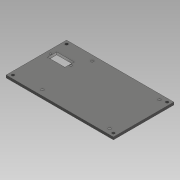
# Autodesk Inventor part: 基本板上
Saved by Autodesk Inventor 2017 (Build 210142000, 142)
## iProperties
Part Number: 基本板上
Material: 一般
Document SubType Name: Modeling
Designer: HISAAKI
Density: 1 g/cm^3
Appearance: 既定
Mass: 37.3682 g
Surface Area: 242.536 cm^2
Volume: 37.3682 cm^3
Author: HISAAKI
Autodesk Inventor part; units mm, degrees
ref_plane "YZ Plane" through (0, 0, 0) normal (1, 0, 0) x (0, 1, 0)
ref_plane "XZ Plane" through (0, 0, 0) normal (0, 1, 0) x (-1, 0, 0)
ref_plane "XY Plane" through (0, 0, 0) normal (0, 0, 1) x (1, 0, 0)
sketch "スケッチ1" plane through (0, 0, 0) normal (0, 0, 1) x (1, 0, 0)
  line L0 (0, 0) -> (142, 0)
  line L1 (142, 0) -> (142, 80)
  line L2 (142, 80) -> (0, 80)
  line L3 (0, 80) -> (0, 0)
  dimension "d40" = 142
  dimension "d41" = 80
  constraints: 8 end point, 2 parallel, 1 horizontal, 1 perpendicular
  measures "d40" distance of L2.end L1.end
  measures "d41" distance of L1.end L0.end
extrude "押し出し1" add sketch "スケッチ1" along normal blind 3.3
hole "穴5" at (4.5, 75.5, 3.3) direction (0, 0, -1) diameter 3.4 end through all
hole "穴6" at (137.5, 75.5, 3.3) direction (0, 0, -1) diameter 3.4 end through all
hole "穴7" at (137.5, 4.5, 3.3) direction (0, 0, -1) diameter 3.4 end through all
hole "穴8" at (4.5, 4.5, 3.3) direction (0, 0, -1) diameter 3.4 end through all
hole "穴9" at (130, 73, 3.3) direction (0, 0, -1) diameter 3.4 end through all
hole "穴10" at (130, 7, 3.3) direction (0, 0, -1) diameter 3.4 end through all
hole "穴13" at (41, 73, 3.3) direction (0, 0, -1) diameter 3.4 end through all
hole "穴14" at (41, 7, 3.3) direction (0, 0, -1) diameter 3.4 end through all
sketch "スケッチ2" plane through (0, 0, 3.3) normal (0, 0, 1) x (1, 0, 0)
  line L0 (7, 60) -> (30, 60)
  line L1 (30, 60) -> (30, 47.8)
  line L2 (30, 47.8) -> (7, 47.8)
  line L3 (7, 47.8) -> (7, 60)
  point P0 (0, 0)
  dimension "d132" = 23
  dimension "d133" = 12.2
  constraints: 8 end point, 2 parallel, 1 horizontal, 1 perpendicular
  measures "d132" distance of L1.end L2.end
  measures "d133" distance of L0.end L1.end
extrude "押し出し2" cut sketch "スケッチ2" against normal blind 10
hole "穴15" at (5, 53.9, 3.3) direction (0, 0, -1) diameter 2.4 end through all
hole "穴16" at (32, 53.9, 3.3) direction (0, 0, -1) diameter 2.4 end through all
